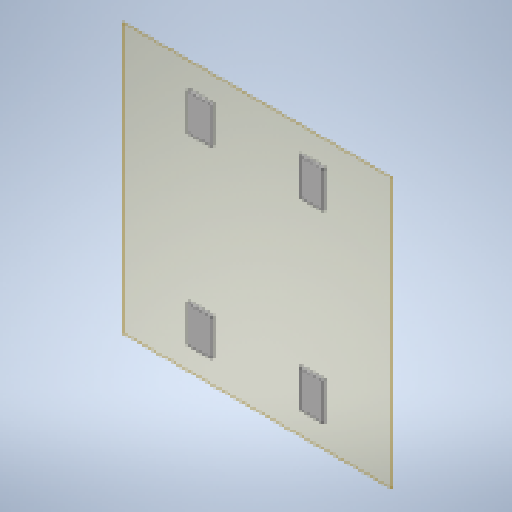
# Autodesk Inventor part: BaseMotor
Saved by Autodesk Inventor 2024 (Build 280153000, 153)
## iProperties
Created: 2025-04-14
Part Number: BaseMotor
Material: Genérico
Document SubType Name: Modeling
Designer: piero
Density: 1 g/cm^3
Appearance: Valor por defecto
Author: piero
Autodesk Inventor part; units mm, degrees
ref_plane "YZ Plane" through (0, 0, 0) normal (1, 0, 0) x (0, 1, 0)
ref_plane "XZ Plane" through (0, 0, 0) normal (0, 1, 0) x (-1, 0, 0)
ref_plane "XY Plane" through (0, 0, 0) normal (0, 0, 1) x (1, 0, 0)
ref_plane "Plano de trabajo1" through (0, 0, 0) normal (0, 0, 1) x (1, 0, 0)
sketch "Boceto1" plane through (0, 0, 0) normal (0, 0, 1) x (1, 0, 0)
  line L0 (-296.2443, -449.783) -> (-296.2443, -299.783) projected
  line L1 (-296.2443, 300.217) -> (-296.2443, 450.217) projected
  line L2 (303.7557, 450.217) -> (303.7557, 300.217) projected
  line L3 (303.7557, -299.783) -> (303.7557, -449.783) projected
  line L4 (-276.2443, -449.783) -> (-176.2443, -449.783)
  line L5 (-176.2443, -449.783) -> (-176.2443, -299.783)
  line L6 (-176.2443, -299.783) -> (-276.2443, -299.783)
  line L7 (-276.2443, -299.783) -> (-276.2443, -449.783)
  line L8 (280, -449.783) -> (180, -449.783)
  line L9 (180, -449.783) -> (180, -299.783)
  line L10 (180, -299.783) -> (280, -299.783)
  line L11 (280, -299.783) -> (280, -449.783)
  line L12 (-276.2443, 450.217) -> (-176.2443, 450.217)
  line L13 (-176.2443, 450.217) -> (-176.2443, 300.217)
  line L14 (-176.2443, 300.217) -> (-276.2443, 300.217)
  line L15 (-276.2443, 300.217) -> (-276.2443, 450.217)
  line L16 (280, 450.217) -> (180, 450.217)
  line L17 (180, 450.217) -> (180, 300.217)
  line L18 (180, 300.217) -> (280, 300.217)
  line L19 (280, 300.217) -> (280, 450.217)
  line L20 (300, -450) -> (300, -300) projected
  line L21 (300, 300) -> (300, 450) projected
  point P0 (0, 0)
  dimension "d0" = 100
  dimension "d1" = 100
  dimension "d2" = 100
  dimension "d3" = 100
  dimension "d4" = 20
  dimension "d5" = 20
  dimension "d6" = 20
  constraints: 32 end point, 8 parallel, 5 point on line, 4 horizontal, 4 perpendicular
  measures "d0" distance of L6.end L5.end
  measures "d1" distance of L9.end L10.end
  measures "d2" distance of L13.end L14.end
  measures "d3" distance of L18.end L17.end
  measures "d4" distance between parallel lines of L15 L1
  measures "d5" distance between parallel lines of L19 L21
  measures "d6" distance between parallel lines of L11 L20
extrude "Extrusión1" add sketch "Boceto1" along normal blind 10
